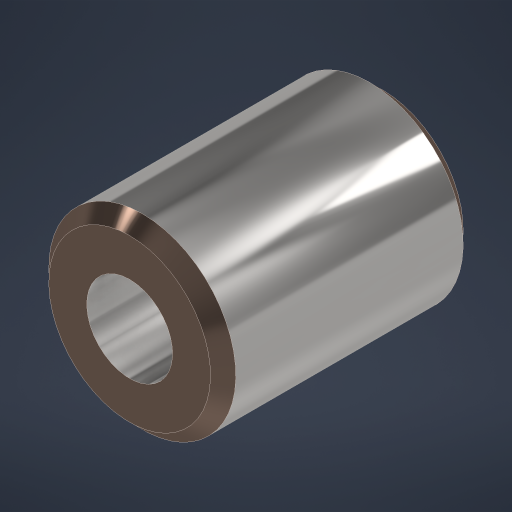
# Autodesk Inventor part: Roller
Saved by Autodesk Inventor 2023 (Build 270158000, 158)
## iProperties
Created: 2022-11-29
Part Number: Roller
Material: Steel
Document SubType Name: Modeling
Designer: iusti
Density: 7.85 g/cm^3
Appearance: Gunmetal - Antique Polished
Author: iusti
Autodesk Inventor part; units mm, degrees
ref_plane "YZ Plane" through (0, 0, 0) normal (1, 0, 0) x (0, 1, 0)
ref_plane "XZ Plane" through (0, 0, 0) normal (0, 1, 0) x (-1, 0, 0)
ref_plane "XY Plane" through (0, 0, 0) normal (0, 0, 1) x (1, 0, 0)
sketch "Sketch1" plane through (0, 0, 0) normal (1, 0, 0) x (0, 1, 0)
  line L0 (3.7, 5) -> (1.7, 5)
  line L1 (1.7, 5) -> (1.7, -5)
  line L2 (1.7, -5) -> (3.7, -5)
  line L3 (3.7, -5) -> (3.7, 5)
  line L4 (0, 5) -> (0, -5)
  point P0 (0, 0)
  point P1 (0, 0)
  dimension "d0" = 10
  dimension "d1" = 3.4
  dimension "d2" = 7.4
  constraints: 10 end point, 2 parallel, 2 point on line, 1 coincident, 1 horizontal, 1 midpoint, 1 perpendicular, 1 vertical
  measures "d0" distance of L2.end L0.start
  measures "d1" diameter of L1 L4
  measures "d2" diameter of L3 L4
revolve "Revolution1" add sketch "Sketch1" angle 360 about axis through (0, 0, 5) along (0, 0, -1)
chamfer "Chamfer1" distance 0.5 angle 45 2 edges at (0, -3.7, 5) (0, -3.7, -5)
body "Solid1"
